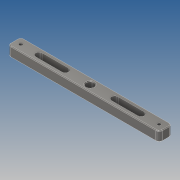
# Autodesk Inventor part: 200-60-DIFFERENTIAL-CONNECTOR-01
Saved by Autodesk Inventor 2018.2 (Build 222227000, 227)
## iProperties
Manager: feesmrt
Company: FRANC0R
Created: 2017-12-05
Part Number: 200-60-DIFFERENTIAL-CONNECTOR-01
Material: Edelstahl
Document SubType Name: Modeling
Designer: feesmrt
Density: 8 g/cm^3
Appearance: Halbpoliert
Project: Rescue Robot
Cost Center: -
Engineer: feesmrt
Authority: feesmrt
Description: Differential Bearing Connector
Stock Number: 200-60-DIFFERENTIAL-CONNECTOR-01
Mass: 288.084 g
Surface Area: 258.81 cm^2
Volume: 106.698 cm^3
Author: feesmrt
Subject: Rescue Robot
Title: Differential Bearing Connector
Revision Number: 1
Autodesk Inventor part; units mm, degrees
ref_plane "YZ Plane" through (0, 0, 0) normal (1, 0, 0) x (0, 1, 0)
ref_plane "XZ Plane" through (0, 0, 0) normal (0, 1, 0) x (-1, 0, 0)
ref_plane "XY Plane" through (0, 0, 0) normal (0, 0, 1) x (1, 0, 0)
sketch "Skizze1" plane through (0, 0, 0) normal (0, 0, 1) x (1, 0, 0)
  line L0 (-161, 0) -> (161, 0) construction
  line L1 (0, 14) -> (0, -14) construction
  line L2 (-115, -10) -> (115, -10)
  line L3 (115, -10) -> (115, 10)
  line L4 (115, 10) -> (-115, 10)
  line L5 (-115, 10) -> (-115, -10)
  line L6 (-115, -10) -> (115, 10) construction
  line L7 (115, -10) -> (-115, 10) construction
  point P0 (0, 0)
  dimension "d0" = 230
  dimension "d1" = 20
  constraints: 12 end point, 2 midpoint, 2 parallel, 1 horizontal, 1 perpendicular
  measures "d0" distance of L3.end L4.end
  measures "d1" distance of L2.end L3.end
extrude "Grundkörper" add sketch "Skizze1" along normal mid plane 15
sketch "Skizze3" plane through (0, 0, 7.5) normal (0, 0, 1) x (1, 0, 0)
  line L0 (0, 14) -> (0, -14) construction
  line L1 (-77.5, 5) -> (-37.5, 5)
  line L2 (-32.5, 0) -> (-32.5, 0)
  line L3 (-37.5, -5) -> (-77.5, -5)
  line L4 (-82.5, 0) -> (-82.5, 0)
  line L5 (-161, 0) -> (161, 0) construction
  line L6 (115, 10) -> (-115, 10) projected
  line L7 (0, 10) -> (-115, 10)
  line L8 (-57.5, 10) -> (-57.5, -10) construction
  line L9 (-115, -10) -> (115, -10) construction
  arc A0 (-82.5, 0) -> (-77.5, -5) centre (-77.5, 0) ccw
  arc A1 (-77.5, 5) -> (-82.5, 0) centre (-77.5, 0) ccw
  arc A2 (-32.5, 0) -> (-37.5, 5) centre (-37.5, 0) ccw
  arc A3 (-37.5, -5) -> (-32.5, 0) centre (-37.5, 0) ccw
  point P0 (0, 0)
  point P1 (-82.5, 5)
  point P2 (-32.5, 5)
  dimension "d16" = 10
  dimension "d17" = 50
  dimension "d18" = 5
  constraints: 12 end point, 8 point on circle, 8 tangent, 5 point on line, 4 centre point, 3 equal radius, 2 midpoint, 2 parallel, 1 collinear, 1 horizontal, 1 perpendicular, 1 vertical, 2 other
  measures "d16" distance between parallel lines of L3 L1
  measures "d17" distance of point (-82.5, 5) point (-32.5, 5)
  measures "d18" radius of A0
extrude "Ausschnitt_Gewichtsreduktion" cut sketch "Skizze3" against normal through all
mirror "Spiegeln_Ausschnitt_Gewichtsreduktion" about plane through (0, 0, 0) normal (1, 0, 0) of "Ausschnitt_Gewichtsreduktion"
sketch "Skizze4" plane through (0, 0, 7.5) normal (0, 0, 1) x (1, 0, 0)
  line L0 (0, 14) -> (0, -14) construction
  line L1 (-161, 0) -> (161, 0) construction
  point P0 (0, 0)
  point P1 (0, 0)
  constraints: 1 coincident
hole "12H7_Bohrung" at (0, 0, 7.5) direction (0, 0, -1) diameter 12 end through all
sketch "Skizze7" plane through (0, 0, -7.5) normal (0, 0, -1) x (-1, 0, 0)
  line L0 (0, -14) -> (0, 14) construction
  line L1 (-161, 0) -> (161, 0) construction
  point P0 (0, 0)
  point P1 (105, 0)
  point P2 (-105, 0)
  dimension "d47" = 210
  constraints: 2 point on line, 1 symmetric about line
  measures "d47" distance of point (105, 0) point (-105, 0)
hole "M6_Bohrung" at (-105, 0, -7.5) at (105, 0, -7.5) direction (0, 0, 1) diameter 4.917 end through all thread size "M6x1" class "6H" standard "ISO Metric profile"
fillet "Abrundung" radius 5 4 edges at (-115, 10, 0) (-115, -10, 0) (115, -10, 0) (115, 10, 0)
chamfer "Fase_Allgemein" distance 1 angle 45 16 edges at (0, -10, 7.5) (113.5355, -8.5355, 7.5) (115, 0, 7.5) (113.5355, 8.5355, 7.5) (0, 10, 7.5) (-113.5355, 8.5355, 7.5) (-115, 0, 7.5) (-113.5355, -8.5355, 7.5) (0, -10, -7.5) (-113.5355, -8.5355, -7.5) (-115, 0, -7.5) (-113.5355, 8.5355, -7.5) (0, 10, -7.5) (113.5355, 8.5355, -7.5) (115, 0, -7.5) (113.5355, -8.5355, -7.5)
chamfer "Fase_Bohrung" distance 1 angle 45 2 edges at (0, 6, 7.5) (0, 6, -7.5)
